Autodesk Inventor part; units mm, degrees
(part 2 of 2)
  arc A582 (-20.1441, -3.8033) -> (-20.0662, -4.1951) centre (0, 0) ccw
  arc A583 (-19.7836, -5.372) -> (-19.6752, -5.7565) centre (0, 0) ccw
  arc A584 (-19.3011, -6.9077) -> (-19.1629, -7.2825) centre (0, 0) ccw
  arc A585 (-18.6997, -8.4007) -> (-18.5324, -8.7635) centre (0, 0) ccw
  arc A586 (-17.9829, -9.842) -> (-17.7877, -10.1905) centre (0, 0) ccw
  arc A587 (-17.1553, -11.2226) -> (-16.9334, -11.5547) centre (0, 0) ccw
  arc A588 (-16.2219, -12.534) -> (-15.9746, -12.8477) centre (0, 0) ccw
  arc A589 (-15.1885, -13.7681) -> (-14.9173, -14.0614) centre (0, 0) ccw
  arc A590 (-14.0614, -14.9173) -> (-13.7681, -15.1885) centre (0, 0) ccw
  arc A591 (-12.8477, -15.9746) -> (-12.534, -16.2219) centre (0, 0) ccw
  arc A592 (-11.5547, -16.9334) -> (-11.2226, -17.1553) centre (0, 0) ccw
  arc A593 (-10.1905, -17.7877) -> (-9.842, -17.9829) centre (0, 0) ccw
  arc A594 (-8.7635, -18.5324) -> (-8.4007, -18.6997) centre (0, 0) ccw
  arc A595 (-7.2825, -19.1629) -> (-6.9077, -19.3011) centre (0, 0) ccw
  arc A596 (-5.7565, -19.6752) -> (-5.372, -19.7836) centre (0, 0) ccw
  arc A597 (-4.1951, -20.0662) -> (-3.8033, -20.1441) centre (0, 0) ccw
  arc A598 (-2.6078, -20.3335) -> (-2.2111, -20.3804) centre (0, 0) ccw
  arc A599 (-1.0044, -20.4754) -> (-0.6052, -20.4911) centre (0, 0) ccw
  arc A600 (0.6052, -20.4911) -> (1.0044, -20.4754) centre (0, 0) ccw
  arc A601 (2.2111, -20.3804) -> (2.6078, -20.3335) centre (0, 0) ccw
  arc A602 (3.8033, -20.1441) -> (4.1951, -20.0662) centre (0, 0) ccw
  arc A603 (5.372, -19.7836) -> (5.7565, -19.6752) centre (0, 0) ccw
  arc A604 (6.9077, -19.3011) -> (7.2825, -19.1629) centre (0, 0) ccw
  arc A605 (8.4007, -18.6997) -> (8.7635, -18.5324) centre (0, 0) ccw
  arc A606 (9.842, -17.9829) -> (10.1905, -17.7877) centre (0, 0) ccw
  arc A607 (11.2226, -17.1553) -> (11.5547, -16.9334) centre (0, 0) ccw
  arc A608 (12.534, -16.2219) -> (12.8477, -15.9746) centre (0, 0) ccw
  arc A609 (13.7681, -15.1885) -> (14.0614, -14.9173) centre (0, 0) ccw
  arc A610 (14.9173, -14.0614) -> (15.1885, -13.7681) centre (0, 0) ccw
  arc A611 (15.9746, -12.8477) -> (16.2219, -12.534) centre (0, 0) ccw
  arc A612 (16.9334, -11.5547) -> (17.1553, -11.2226) centre (0, 0) ccw
  arc A613 (17.7877, -10.1905) -> (17.9829, -9.842) centre (0, 0) ccw
  arc A614 (18.5324, -8.7635) -> (18.6997, -8.4007) centre (0, 0) ccw
  arc A615 (19.1629, -7.2825) -> (19.3011, -6.9077) centre (0, 0) ccw
  arc A616 (19.6752, -5.7565) -> (19.7836, -5.372) centre (0, 0) ccw
  arc A617 (20.0662, -4.1951) -> (20.1441, -3.8033) centre (0, 0) ccw
  arc A618 (20.3335, -2.6078) -> (20.3804, -2.2111) centre (0, 0) ccw
  arc A619 (20.4754, -1.0044) -> (20.4911, -0.6052) centre (0, 0) ccw
  arc A620 (20.4911, 0.6052) -> (20.4754, 1.0044) centre (0, 0) ccw
  arc A621 (20.3804, 2.2111) -> (20.3335, 2.6078) centre (0, 0) ccw
  arc A622 (20.1441, 3.8033) -> (20.0662, 4.1951) centre (0, 0) ccw
  arc A623 (19.7836, 5.372) -> (19.6752, 5.7565) centre (0, 0) ccw
  arc A624 (19.3011, 6.9077) -> (19.1629, 7.2825) centre (0, 0) ccw
  arc A625 (18.6997, 8.4007) -> (18.5324, 8.7635) centre (0, 0) ccw
  arc A626 (17.9829, 9.842) -> (17.7877, 10.1905) centre (0, 0) ccw
  arc A627 (17.1553, 11.2226) -> (16.9334, 11.5547) centre (0, 0) ccw
  arc A628 (16.2219, 12.534) -> (15.9746, 12.8477) centre (0, 0) ccw
  arc A629 (15.1885, 13.7681) -> (14.9173, 14.0614) centre (0, 0) ccw
  arc A630 (14.0614, 14.9173) -> (13.7681, 15.1885) centre (0, 0) ccw
  arc A631 (12.8477, 15.9746) -> (12.534, 16.2219) centre (0, 0) ccw
  arc A632 (11.5547, 16.9334) -> (11.2226, 17.1553) centre (0, 0) ccw
  arc A633 (10.1905, 17.7877) -> (9.842, 17.9829) centre (0, 0) ccw
  arc A634 (8.7635, 18.5324) -> (8.4007, 18.6997) centre (0, 0) ccw
  arc A635 (7.2825, 19.1629) -> (6.9077, 19.3011) centre (0, 0) ccw
  arc A636 (5.7565, 19.6752) -> (5.372, 19.7836) centre (0, 0) ccw
  arc A637 (4.1951, 20.0662) -> (3.8033, 20.1441) centre (0, 0) ccw
  arc A638 (2.6078, 20.3335) -> (2.2111, 20.3804) centre (0, 0) ccw
  arc A639 (1.0044, 20.4754) -> (0.6052, 20.4911) centre (0, 0) ccw
  line L0 (-22.5, 0) -> (22.5, 0)
  line L1 (0, -22.5) -> (0, 22.5)
  line L2 (40.5, 20.5) -> (110.5, 20.5)
  line L3 (40.5, 12.5) -> (110.5, 12.5)
  line L4 (40.5, 4.5) -> (110.5, 4.5)
  line L5 (40.5, -3.5) -> (110.5, -3.5)
  line L6 (40.5, -11.5) -> (110.5, -11.5)
  line L7 (40.5, -19.5) -> (110.5, -19.5)
  line L8 (40.5, -27.5) -> (110.5, -27.5)
  line L9 (40.5, -35.5) -> (110.5, -35.5)
  line L10 (40.5, -43.5) -> (110.5, -43.5)
  line L11 (40.5, -51.5) -> (110.5, -51.5)
  line L12 (40.5, -59.5) -> (110.5, -59.5)
  line L13 (40.5, -67.5) -> (110.5, -67.5)
  line L14 (40.5, -75.5) -> (110.5, -75.5)
  line L15 (40.5, 20.5) -> (40.5, -75.5)
  line L16 (110.5, 20.5) -> (110.5, -75.5)
  line L17 (75.5, 12.5) -> (75.5, -75.5)
  point P0 (0, 0)
  point P1 (46.5, 14.5)
  point P2 (49, 6.5)
  point P3 (49, -1.5)
  point P4 (46.5, -9.5)
  point P5 (49, -17.5)
  point P6 (44, -25.5)
  point P7 (46.5, -33.5)
  point P8 (46.5, -41.5)
  point P9 (46.5, -49.5)
  point P10 (49, -57.5)
  point P11 (49, -65.5)
  point P12 (46.5, -73.5)
  point P13 (76.5, 6.5)
  point P14 (91.5, -1.5)
  point P15 (90.25, -9.5)
  point P16 (89, -17.5)
  point P17 (91.5, -25.5)
  point P18 (85.25, -33.5)
  point P19 (91.5, -41.5)
  point P20 (87.75, -49.5)
  point P21 (86.5, -57.5)
  point P22 (94, -65.5)
  point P23 (94, -73.5)
  point P24 (1, 36)
  point P25 (1, 30)
  point P26 (17.1875, 36)
  point P27 (19.3125, 30)
  constraints: 960 point on circle, 480 centre point, 32 end point, 2 horizontal alignment, 2 midpoint, 2 vertical alignment, 504 other
extrude "押し出し2" add sketch "スケッチ4" against normal blind 3 contours A1 A2 A639 A479 A478 A477 A559 A237 A238 A239 A638 A476 A475 A474 A558 A234 A235 A236 A637 A473 A472 A471 A557 A231 A232 A233 A636 A470 A469 A468 A556 A228 A229 A230 A635 A467 A466 A465 A555 A225 A226 A227 A634 A464 A463 A462 A554 A222 A223 A224 A633 A461 A460 A459 A553 A219 A220 A221 A632 A458 A457 A456 A552 A216 A217 A218 A631 A455 A454 A453 A551 A213 A214 A215 A630 A452 A451 A450 A550 A210 A211 A212 A629 A449 A448 A447 A549 A207 A208 A209 A628 A446 A445 A444 A548 A204 A205 A206 A627 A443 A442 A441 A547 A201 A202 A203 A626 A440 A439 A438 A546 A198 A199 A200 A625 A437 A436 A435 A545 A195 A196 A197 A624 A434 A433 A432 A544 A192 A193 A194 A623 A431 A430 A429 A543 A189 A190 A191 A622 A428 A427 A426 A542 A186 A187 A188 A621 A425 A424 A423 A541 A183 A184 A185 A620 A422 A421 A420 A540 L0 L1 A480 A0 | L1 L0 A500 A60 A61 A62 A579 A299 A298 A297 A499 A57 A58 A59 A578 A296 A295 A294 A498 A54 A55 A56 A577 A293 A292 A291 A497 A51 A52 A53 A576 A290 A289 A288 A496 A48 A49 A50 A575 A287 A286 A285 A495 A45 A46 A47 A574 A284 A283 A282 A494 A42 A43 A44 A573 A281 A280 A279 A493 A39 A40 A41 A572 A278 A277 A276 A492 A36 A37 A38 A571 A275 A274 A273 A491 A33 A34 A35 A570 A272 A271 A270 A490 A30 A31 A32 A569 A269 A268 A267 A489 A27 A28 A29 A568 A266 A265 A264 A488 A24 A25 A26 A567 A263 A262 A261 A487 A21 A22 A23 A566 A260 A259 A258 A486 A18 A19 A20 A565 A257 A256 A255 A485 A15 A16 A17 A564 A254 A253 A252 A484 A12 A13 A14 A563 A251 A250 A249 A483 A9 A10 A11 A562 A248 A247 A246 A482 A6 A7 A8 A561 A245 A244 A243 A481 A3 A4 A5 A560 A242 A241 A240 A480 | L1 A520 A120 A121 A122 A599 A359 A358 A357 A519 A117 A118 A119 A598 A356 A355 A354 A518 A114 A115 A116 A597 A353 A352 A351 A517 A111 A112 A113 A596 A350 A349 A348 A516 A108 A109 A110 A595 A347 A346 A345 A515 A105 A106 A107 A594 A344 A343 A342 A514 A102 A103 A104 A593 A341 A340 A339 A513 A99 A100 A101 A592 A338 A337 A336 A512 A96 A97 A98 A591 A335 A334 A333 A511 A93 A94 A95 A590 A332 A331 A330 A510 A90 A91 A92 A589 A329 A328 A327 A509 A87 A88 A89 A588 A326 A325 A324 A508 A84 A85 A86 A587 A323 A322 A321 A507 A81 A82 A83 A586 A320 A319 A318 A506 A78 A79 A80 A585 A317 A316 A315 A505 A75 A76 A77 A584 A314 A313 A312 A504 A72 A73 A74 A583 A311 A310 A309 A503 A69 A70 A71 A582 A308 A307 A306 A502 A66 A67 A68 A581 A305 A304 A303 A501 A63 A64 A65 A580 A302 A301 A300 A500 L0 | L0 A540 A180 A181 A182 A619 A419 A418 A417 A539 A177 A178 A179 A618 A416 A415 A414 A538 A174 A175 A176 A617 A413 A412 A411 A537 A171 A172 A173 A616 A410 A409 A408 A536 A168 A169 A170 A615 A407 A406 A405 A535 A165 A166 A167 A614 A404 A403 A402 A534 A162 A163 A164 A613 A401 A400 A399 A533 A159 A160 A161 A612 A398 A397 A396 A532 A156 A157 A158 A611 A395 A394 A393 A531 A153 A154 A155 A610 A392 A391 A390 A530 A150 A151 A152 A609 A389 A388 A387 A529 A147 A148 A149 A608 A386 A385 A384 A528 A144 A145 A146 A607 A383 A382 A381 A527 A141 A142 A143 A606 A380 A379 A378 A526 A138 A139 A140 A605 A377 A376 A375 A525 A135 A136 A137 A604 A374 A373 A372 A524 A132 A133 A134 A603 A371 A370 A369 A523 A129 A130 A131 A602 A368 A367 A366 A522 A126 A127 A128 A601 A365 A364 A363 A521 A123 A124 A125 A600 A362 A361 A360 A520 L1
sketch "スケッチ7" plane through (0, 0, 0) normal (0, 0, -1) x (-1, 0, 0)
  circle A0 centre (0, 0) radius 18.25
  dimension "d97" = 36.5
  constraints: 1 centre point, 1 coincident
  measures "d97" diameter of A0
extrude "押し出し7" cut sketch "スケッチ7" against normal blind 0.75
sketch "スケッチ8" plane through (0, 0, 3) normal (0, 0, 1) x (1, 0, 0)
  circle A0 centre (0, 0) radius 18.25
  dimension "d100" = 36.5
  constraints: 1 centre point, 1 coincident
  measures "d100" diameter of A0
extrude "押し出し8" cut sketch "スケッチ8" against normal blind 0.75
sketch "スケッチ9" plane through (0, 0, 2.25) normal (0, 0, 1) x (1, 0, 0)
  circle A0 centre (0, 0) radius 6
  circle A1 centre (0, 0) radius 11.5
  line L0 (-6.612, 6.3969) -> (-0.1521, 9.1987) construction
  line L1 (-0.1521, 9.1987) -> (6.3969, 6.612) construction
  line L2 (6.3969, 6.612) -> (9.1987, 0.1521) construction
  line L3 (9.1987, 0.1521) -> (6.612, -6.3969) construction
  line L4 (6.612, -6.3969) -> (0.1521, -9.1987) construction
  line L5 (0.1521, -9.1987) -> (-6.3969, -6.612) construction
  line L6 (-6.3969, -6.612) -> (-9.1987, -0.1521) construction
  line L7 (-9.1987, -0.1521) -> (-6.612, 6.3969) construction
  circle A2 centre (-6.612, 6.3969) radius 1.5
  circle A3 centre (-6.612, 6.3969) radius 3 construction
  circle A4 centre (-0.1521, 9.1987) radius 3 construction
  circle A5 centre (-0.1521, 9.1987) radius 1.5
  circle A6 centre (6.3969, 6.612) radius 1.5
  circle A7 centre (9.1987, 0.1521) radius 1.5
  circle A8 centre (6.612, -6.3969) radius 1.5
  circle A9 centre (0.1521, -9.1987) radius 1.5
  circle A10 centre (-6.3969, -6.612) radius 1.5
  circle A11 centre (-9.1987, -0.1521) radius 1.5
  dimension "d103" = 12
  dimension "d104" = 23
  dimension "d105" = 3
  dimension "d106" = 6
  dimension "d107" = 6
  dimension "d108" = 3
  dimension "d109" = 3
  dimension "d110" = 3
  dimension "d111" = 3
  dimension "d112" = 3
  dimension "d113" = 3
  dimension "d114" = 3
  dimension "d115" = 9.2
  constraints: 16 end point, 13 coincident, 12 centre point, 17 other
  measures "d103" diameter of A0
  measures "d104" diameter of A1
  measures "d105" diameter of A2
  measures "d106" diameter of A3
  measures "d107" diameter of A4
  measures "d108" diameter of A5
  measures "d109" diameter of A6
  measures "d110" diameter of A7
  measures "d111" diameter of A8
  measures "d112" diameter of A9
  measures "d113" diameter of A10
  measures "d114" diameter of A11
  measures "d115" distance of point (0, 0) L6.end
sketch "スケッチ10" plane through (0, 0, 2.25) normal (0, 0, 1) x (1, 0, 0)
  circle A0 centre (0, 0) radius 17.5
  circle A1 centre (0, 0) radius 15 construction
  circle A2 centre (-0.0185, 15) radius 1.5
  arc A3 (1.3802, 16.4422) -> (-1.3922, 16.4412) centre (0, 0) ccw
  arc A4 (15.2271, 6.3549) -> (1.3802, 16.4422) centre (0, 0) ccw
  arc A5 (-1.3922, 16.4412) -> (-15.5317, 5.5691) centre (0, 0) ccw
  arc A6 (-15.7143, -5.031) -> (-7.6771, -14.6052) centre (0, 0) ccw
  arc A7 (-7.6771, -14.6052) -> (3.9215, -16.0272) centre (0, 0) ccw
  arc A8 (3.9215, -16.0272) -> (14.9167, -7.0527) centre (0, 0) ccw
  arc A9 (-15.5317, 5.5691) -> (-15.7143, -5.031) centre (0, 0) ccw
  arc A10 (14.9167, -7.0527) -> (15.2271, 6.3549) centre (0, 0) ccw
  circle A11 centre (-0.0185, 15) radius 1.25 construction
  circle A12 centre (-6.525, 13.5065) radius 1.5
  circle A13 centre (-6.525, 13.5065) radius 1.25 construction
  circle A14 centre (-11.739, 9.3378) radius 1.5
  circle A15 centre (-11.739, 9.3378) radius 1.25 construction
  circle A16 centre (-14.628, 3.3197) radius 1.5
  circle A17 centre (-14.628, 3.3197) radius 1.25 construction
  circle A18 centre (-14.6198, -3.3559) radius 1.5
  circle A19 centre (-14.6198, -3.3559) radius 1.25 construction
  circle A20 centre (-11.7159, -9.3668) radius 1.5
  circle A21 centre (-11.7159, -9.3668) radius 1.25 construction
  circle A22 centre (-6.4915, -13.5226) radius 1.5
  circle A23 centre (-6.4915, -13.5226) radius 1.25 construction
  circle A24 centre (0.0185, -15) radius 1.5
  circle A25 centre (0.0185, -15) radius 1.25 construction
  circle A26 centre (6.525, -13.5065) radius 1.5
  circle A27 centre (6.525, -13.5065) radius 1.25 construction
  circle A28 centre (11.739, -9.3378) radius 1.5
  circle A29 centre (11.739, -9.3378) radius 1.25 construction
  circle A30 centre (14.628, -3.3197) radius 1.5
  circle A31 centre (14.628, -3.3197) radius 1.25 construction
  circle A32 centre (14.6198, 3.3559) radius 1.5
  circle A33 centre (14.6198, 3.3559) radius 1.25 construction
  circle A34 centre (11.7159, 9.3668) radius 1.5
  circle A35 centre (11.7159, 9.3668) radius 1.25 construction
  circle A36 centre (6.4915, 13.5226) radius 1.5
  circle A37 centre (6.4915, 13.5226) radius 1.25 construction
  dimension "d119" = 30
  dimension "d118" = 35
  dimension "d120" = 3
  dimension "d121" = 33
  dimension "d122" = 2.5
  dimension "d137" = 360
  constraints: 37 centre point, 19 coincident, 16 point on circle, 60 other
  measures "d118" diameter of A0
  measures "d120" diameter of A2
  measures "d121" diameter of A3
  measures "d122" diameter of A11
extrude "押し出し9" cut sketch "スケッチ10" against normal blind 3 contours A2 | A14 | A16 | A20 | A24 | A28 | A30 | A34
sketch "スケッチ11" plane through (0, 0, 2.25) normal (0, 0, 1) x (1, 0, 0)
  circle A0 centre (0, 0) radius 8
  dimension "d141" = 16
  constraints: 1 centre point, 1 coincident
  measures "d141" diameter of A0
extrude "押し出し10" cut sketch "スケッチ11" against normal blind 3
sketch "スケッチ12" plane through (0, 0, 2.25) normal (0, 0, 1) x (1, 0, 0)
  circle A0 centre (0, 0) radius 8 projected
  circle A1 centre (14.628, -3.3197) radius 1.5 projected
  circle A2 centre (0.0185, -15) radius 1.5 projected
  circle A3 centre (-14.628, 3.3197) radius 1.5 projected
  circle A4 centre (-0.0185, 15) radius 1.5 projected
  circle A5 centre (-11.739, 9.3378) radius 1.5 projected
  circle A6 centre (-11.7159, -9.3668) radius 1.5 projected
  circle A7 centre (11.739, -9.3378) radius 1.5 projected
  circle A8 centre (11.7159, 9.3668) radius 1.5 projected
  circle A9 centre (0, 0) radius 18.25 projected
sketch "スケッチ13" plane through (0, 0, 2.25) normal (0, 0, 1) x (1, 0, 0)
  circle A0 centre (0, 0) radius 18.25 projected
  circle A1 centre (26.1722, 2.1655) radius 1.9507
  constraints: 1 centre point
extrude "押し出し11" add sketch "スケッチ13" against normal blind 1.5 contours A0
sketch "スケッチ17" plane through (0, 0, 2.25) normal (0, 0, 1) x (1, 0, 0)
  circle A0 centre (0, 0) radius 2
  dimension "d152" = 4
  constraints: 1 centre point, 1 coincident
  measures "d152" diameter of A0
extrude "押し出し14" cut sketch "スケッチ17" against normal blind 10
sketch "スケッチ19" plane through (0, 0, 2.25) normal (0, 0, 1) x (1, 0, 0)
  circle A0 centre (0, 0) radius 9
  dimension "d161" = 18
  constraints: 1 centre point, 1 coincident
  measures "d161" diameter of A0
extrude "押し出し16" cut sketch "スケッチ19" against normal blind 10
sketch "スケッチ21" plane through (0, 0, 2.25) normal (0, 0, 1) x (1, 0, 0)
  circle A0 centre (0, 0) radius 14.5 construction
  line L0 (0, 0) -> (0, 14.5) construction
  line L1 (0, 0) -> (-12.5574, -7.25) construction
  line L2 (0, 0) -> (12.5574, -7.25) construction
  circle A1 centre (0, 14.5) radius 1.5
  circle A2 centre (-12.5574, -7.25) radius 1.5
  circle A3 centre (12.5574, -7.25) radius 1.5
  dimension "d164" = 29
  dimension "d165" = 120
  dimension "d166" = 120
  dimension "d167" = 3
  dimension "d168" = 3
  dimension "d169" = 3
  constraints: 6 end point, 4 centre point, 4 coincident, 3 point on circle, 1 vertical
  measures "d164" diameter of A0
  measures "d165" angle of L2 L0
  measures "d166" angle of L0 L1
  measures "d167" diameter of A1
  measures "d168" diameter of A2
  measures "d169" diameter of A3
extrude "押し出し18" cut sketch "スケッチ21" against normal blind 3
sketch "スケッチ22" plane through (0, 0, 2.25) normal (0, 0, 1) x (1, 0, 0)
  circle A0 centre (-12.5574, -7.25) radius 1.5 projected
  circle A1 centre (0, 14.5) radius 1.5 projected
  circle A2 centre (12.5574, -7.25) radius 1.5 projected
  circle A3 centre (0, 0) radius 9 projected
  circle A4 centre (0, 0) radius 18.25 projected
  circle A5 centre (0, 0) radius 12 construction
  circle A6 centre (0, 0) radius 16.25 construction
  line L0 (0, 0) -> (14.0729, 8.125) construction
  line L1 (0, 0) -> (0, -16.25) construction
  line L2 (0, 0) -> (-14.0729, 8.125) construction
  circle A7 centre (-12.2326, 7.0625) radius 2.125
  circle A8 centre (12.2326, 7.0625) radius 2.125
  circle A9 centre (0, -14.125) radius 2.125
  dimension "d174" = 3
  dimension "d175" = 2
  dimension "d176" = 120
  dimension "d177" = 120
  dimension "d182" = 32.5
  constraints: 6 end point, 6 tangent, 5 centre point, 3 point on circle, 3 point on line, 1 vertical
  measures "d174" radial gap between concentric circles of A3 A5
  measures "d175" radial gap between concentric circles of A4 A6
  measures "d176" angle of L1 L0
  measures "d177" angle of L1 L2
  measures "d182" diameter of A6
extrude "押し出し19" cut sketch "スケッチ22" against normal blind 3 contours A7 | A8 | A9
sketch "スケッチ25" plane through (0, 0, 2.25) normal (0, 0, 1) x (1, 0, 0)
  circle A0 centre (12.2326, 7.0625) radius 2.125 construction
  circle A1 centre (-12.2326, 7.0625) radius 2.125 construction
  circle A2 centre (0, -14.125) radius 2.125 construction
  circle A3 centre (-12.5574, -7.25) radius 1.5 projected
  circle A4 centre (0, 14.5) radius 1.5 projected
  circle A5 centre (12.5574, -7.25) radius 1.5 projected
  circle A6 centre (0, 0) radius 9 projected
  circle A7 centre (0, 0) radius 18.25 projected
  arc A8 (2.7825, 18.0366) -> (4.4994, 14.5711) centre (0, 14.5) ccw
  arc A9 (-13.822, -6.4433) -> (-12.491, -8.7485) centre (0, 0) ccw
  arc A10 (-17.0114, -6.6086) -> (-14.2289, -11.428) centre (-12.5574, -7.25) ccw
  arc A11 (-10.3692, -11.1822) -> (-14.8687, -3.3889) centre (-12.5574, -7.25) ccw
  arc A12 (-10.3692, -11.1822) -> (10.3692, -11.1822) centre (0, 0) ccw
  arc A13 (12.491, -8.7485) -> (13.822, -6.4433) centre (0, 0) ccw
  arc A14 (14.8687, -3.3889) -> (10.3692, -11.1822) centre (12.5574, -7.25) ccw
  arc A15 (14.2289, -11.428) -> (17.0114, -6.6086) centre (12.5574, -7.25) ccw
  arc A16 (14.8687, -3.3889) -> (4.4994, 14.5711) centre (0, 0) ccw
  arc A17 (1.3309, 15.1918) -> (-1.3309, 15.1918) centre (0, 0) ccw
  arc A18 (-4.4994, 14.5711) -> (-14.8687, -3.3889) centre (0, 0) ccw
  dimension "d184" = 3
  constraints: 34 point on circle, 11 centre point
  measures "d184" radial gap between concentric circles of A4 A8
extrude "押し出し20" cut sketch "スケッチ25" against normal blind 10 contours A8 A16 A14 A12 A11 A18
sketch "スケッチ26" plane through (0, 0, 2.25) normal (0, 0, 1) x (1, 0, 0)
  arc A0 (-12.1724, 9.1866) -> (-14.0421, 5.9483) centre (-12.2326, 7.0625) ccw projected
  arc A1 (-1.8697, -15.135) -> (1.8697, -15.135) centre (0, -14.125) ccw projected
  arc A2 (14.0421, 5.9483) -> (12.1724, 9.1866) centre (12.2326, 7.0625) ccw projected
  arc A3 (-12.1724, 9.1866) -> (-14.0421, 5.9483) centre (0, 0) ccw
  arc A4 (-1.8697, -15.135) -> (1.8697, -15.135) centre (0, 0) ccw
  arc A5 (14.0421, 5.9483) -> (12.1724, 9.1866) centre (12.2326, 7.0625) ccw projected
  arc A6 (14.0421, 5.9483) -> (12.1724, 9.1866) centre (0, 0) ccw
  constraints: 8 point on circle, 3 centre point, 3 coincident
extrude "押し出し21" add sketch "スケッチ26" against normal blind 1.5
fillet "フィレット1" radius 4 6 edges at (10.3692, -11.1822, 1.5) (-10.3692, -11.1822, 1.5) (-14.8687, -3.3889, 1.5) (4.4994, 14.5711, 1.5) (-4.4994, 14.5711, 1.5) (14.8687, -3.3889, 1.5)
